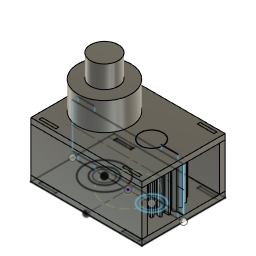
Dual Rotary Encoder Proto (Autodesk Fusion 360 design; units mm, degrees)
description: Spur Gear; Module: 0.7083333333333334; Num Teeth: 24; Pressure Angle: 20.0; Backlash: 0.00 mm
Autodesk Fusion 360 part; units mm, degrees
note: some values were not read from the file. Set by a fixed rule: which sketch regions a step uses.
sketch "BasePlate" plane through (0, 0, 0) normal (0, 0, 1) x (1, 0, 0)
  line L0 (-20, 15) -> (20, 15)
  line L1 (20, 15) -> (20, -15)
  line L2 (20, -15) -> (-20, -15)
  line L3 (-20, -15) -> (-20, 15)
  line L4 (0, 0) -> (-8.5, 0) construction
  line L5 (0, 0) -> (8.5, 0) construction
  circle A0 centre (-8.5, 0) radius 4.125
  circle A1 centre (8.5, 0) radius 4.125
  circle A2 centre (-8.5, 0) radius 7
  line L6 (-18, 14) -> (-12, 14)
  line L7 (-12, 14) -> (-12, 13)
  line L8 (-12, 13) -> (-18, 13)
  line L9 (-18, 13) -> (-18, 14)
  line L10 (18, 14) -> (12, 14)
  line L11 (12, 14) -> (12, 13)
  line L12 (12, 13) -> (18, 13)
  line L13 (18, 13) -> (18, 14)
  line L14 (18, -13) -> (12, -13)
  line L15 (12, -13) -> (12, -14)
  line L16 (12, -14) -> (18, -14)
  line L17 (18, -14) -> (18, -13)
  line L18 (-18, -13) -> (-12, -13)
  line L19 (-12, -13) -> (-12, -14)
  line L20 (-12, -14) -> (-18, -14)
  line L21 (-18, -14) -> (-18, -13)
  line L22 (-18, 13) -> (-20, 13) construction
  line L23 (-12, 14) -> (-12, 15) construction
  line L24 (12, 14) -> (12, 15) construction
  line L25 (18, 13) -> (20, 13) construction
  line L26 (-18, -13) -> (-20, -13) construction
  line L27 (-12, -14) -> (-12, -15) construction
  line L28 (12, -14) -> (12, -15) construction
  line L29 (18, -13) -> (20, -13) construction
  line L30 (0, 15) -> (0, -15)
  circle A3 centre (-8.5, 0) radius 3
  circle A4 centre (8.5, 0) radius 3
  circle A5 centre (8.5, 0) radius 4
  circle A6 centre (-8.5, 0) radius 4
  line L31 (-20, 0) -> (20, 0)
  circle A7 centre (-8.5, 0) radius 7.125
  line L32 (-17.85, 13.85) -> (-12.15, 13.85)
  line L33 (-12.15, 13.85) -> (-12.15, 13.15)
  line L34 (-12.15, 13.15) -> (-17.85, 13.15)
  line L35 (-17.85, 13.15) -> (-17.85, 13.85)
  dimension "d1" = 8.5
  dimension "d3" = 8.5
  dimension "d5" = 8.25
  dimension "d8" = 14
  dimension "d14" = 6
  dimension "d15" = 2
  dimension "d16" = 40
  dimension "d20" = 30
  dimension "d23" = 6
  dimension "d24" = 8
  dimension "d26" = 1
  dimension "d27" = 1
  dimension "d56" = 14.25
  dimension "d79" = 0.15
  constraint horizontal L0
  constraint vertical L1
  constraint horizontal L2
  constraint vertical L3
  constraint coincident L4.start L5.start
  constraint horizontal L4
  constraint coincident L4.end A0.centre
  constraint coincident L5.end A1.centre
  constraint concentric A0 A2
  constraint horizontal L6
  constraint vertical L7
  constraint horizontal L8
  constraint vertical L9
  constraint horizontal L10
  constraint vertical L11
  constraint horizontal L12
  constraint vertical L13
  constraint horizontal L14
  constraint vertical L15
  constraint horizontal L16
  constraint vertical L17
  constraint horizontal L18
  constraint vertical L19
  constraint horizontal L20
  constraint vertical L21
  constraint coincident L3 L22.end
  constraint perpendicular L3 L22
  constraint coincident L0 L23.end
  constraint perpendicular L0 L23
  constraint coincident L0 L24.end
  constraint perpendicular L0 L24
  constraint perpendicular L13 L25
  constraint coincident L3 L26.end
  constraint perpendicular L3 L26
  constraint coincident L2 L27.end
  constraint perpendicular L2 L27
  constraint coincident L2 L28.end
  constraint perpendicular L2 L28
  constraint coincident L1 L29.end
  constraint perpendicular L1 L29
  constraint coincident L0 L30.start
  constraint perpendicular L0 L30
  constraint midpoint L0 L30.start
  constraint midpoint L4.start L30
  constraint concentric A0 A3
  constraint concentric A1 A4
  constraint concentric A1 A5
  constraint concentric A0 A6
  constraint coincident L1 L25.end
  constraint equal A0 A1
  constraint equal A5 A6
  constraint equal A3 A4
  constraint equal L22 L25
  constraint equal L23 L24
  constraint equal L8 L12
  constraint midpoint L3 L31.start
  constraint midpoint L1 L31.end
  constraint midpoint L4.start L31
  constraint equal L22 L26
  constraint equal L8 L18
  constraint equal L7 L19
  constraint equal L23 L27
  constraint equal L7 L11
  constraint equal L7 L15
  constraint equal L23 L28
  constraint equal L8 L14
  constraint equal L22 L29
  constraint concentric A3 A7
  measures "d1" distance of L4.start L4.end
  measures "d3" distance of L4.start L5.end
  measures "d5" diameter of A1
  measures "d8" diameter of A2
  measures "d14" distance of L7.end L8.end
  measures "d15" distance of L8.end L22.end
  measures "d16" distance of L0.start L0.end
  measures "d20" distance of L0.start L2.end
  measures "d23" diameter of A4
  measures "d24" diameter of A5
  measures "d26" distance of L6.end L7.end
  measures "d27" distance of L6.end L23.end
  measures "d56" diameter of A7
extrude "Extrude1" add sketch "BasePlate" along normal blind 2 contours L0 L3 L30 L31 A7 | L0 L1 A1 L30 L31 | L2 L3 L30 L31 A7 | L1 L2 A1 L30 L31 | A2 L31 A7 | A2 L31 A7 | A0 A2 L31 | A0 A2 L31 makes body 1 in component "Panel Bottom"
extrude "Extrude1'" add sketch "BasePlate" along normal blind 2 separate body contours L0 L3 L30 L31 A7 | L0 L1 A1 L30 L31 | L2 L3 L30 L31 A7 | L1 L2 A1 L30 L31 makes body 2 in component "Panel Top"
move_body "Move1" bodies 2 to x (1, 0, 0) y (0, 1, 0) z (0, 0, 1) at (0, 0, 18) in component "Panel Top"
extrude "Extrude1''" add sketch "BasePlate" along normal blind 20 separate body contours A4 A5 L31 | A4 A5 L31 | A4 L31 | A4 L31 makes body 3 in component "Axle Coarse"
extrude "Extrude2" cut sketch "BasePlate" along normal blind 6 contours A4 L31 | A4 L31 bodies 3 in component "Axle Coarse"
sketch "Sketch1" plane through (0, 0, 0) normal (0, 0, 1) x (1, 0, 0) in component "Spur Gear (24 teeth)"
  circle A0 centre (0, 0) radius 7.5992
  circle A1 centre (0, 0) radius 3
extrude "Extrude1'''" add sketch "Sketch1" along normal blind 16 separate body makes body 4 in component "Spur Gear (24 teeth)"
sketch "Sketch2" plane through (0, 0, 0) normal (0, 0, 1) x (1, 0, 0) in component "Spur Gear (24 teeth)"
  spline S0 degree 5 poles (7.9616, -0.6411) (7.9652, -0.6414) (7.9722, -0.6419) (7.9828, -0.6423) (7.997, -0.6424) (8.0148, -0.6419) (8.0325, -0.6408) (8.0503, -0.6395) (8.0681, -0.6379) (8.086, -0.6363) (8.1038, -0.6345) (8.1216, -0.6326) (8.1395, -0.6304) (8.1573, -0.628) (8.1752, -0.6254) (8.193, -0.6226) (8.2109, -0.6196) (8.2287, -0.6163) (8.2466, -0.613) (8.2645, -0.6095) (8.2823, -0.6059) (8.3002, -0.6022) (8.3181, -0.5983) (8.336, -0.5942) (8.3538, -0.59) (8.3717, -0.5856) (8.3896, -0.5812) (8.4074, -0.5765) (8.4253, -0.5718) (8.4432, -0.5669) (8.461, -0.5619) (8.4789, -0.5568) (8.4968, -0.5516) (8.5146, -0.5462) (8.5325, -0.5407) (8.5503, -0.5351) (8.5681, -0.5294) (8.586, -0.5235) (8.6038, -0.5176) (8.6216, -0.5115) (8.6394, -0.5053) (8.6573, -0.499) (8.6751, -0.4926) (8.6929, -0.4861) (8.7107, -0.4795) (8.7284, -0.4728) (8.7462, -0.4659) (8.764, -0.459) (8.7817, -0.452) (8.7995, -0.4448) (8.8172, -0.4376) (8.835, -0.4302) (8.8527, -0.4228) (8.8704, -0.4152) (8.8881, -0.4076) (8.9058, -0.3998) (8.9235, -0.392) (8.9412, -0.384) (8.9588, -0.376) (8.9765, -0.3678) (8.9941, -0.3596) (9.0118, -0.3513) (9.0294, -0.3428) (9.047, -0.3343) (9.0646, -0.3257) (9.0822, -0.317) (9.0997, -0.3082) (9.1173, -0.2993) (9.1348, -0.2903) (9.1523, -0.2812) (9.1699, -0.272) (9.1839, -0.2646) (9.1944, -0.259) (9.2014, -0.2553) (9.2048, -0.2534) knots 0 0 0 0 0 0 0.01428571 0.02857143 0.04285714 0.05714286 0.07142857 0.08571429 0.1 0.11428571 0.12857143 0.14285714 0.15714286 0.17142857 0.18571429 0.2 0.21428571 0.22857143 0.24285714 0.25714286 0.27142857 0.28571429 0.3 0.31428571 0.32857143 0.34285714 0.35714286 0.37142857 0.38571429 0.4 0.41428571 0.42857143 0.44285714 0.45714286 0.47142857 0.48571429 0.5 0.51428571 0.52857143 0.54285714 0.55714286 0.57142857 0.58571429 0.6 0.61428571 0.62857143 0.64285714 0.65714286 0.67142857 0.68571429 0.7 0.71428571 0.72857143 0.74285714 0.75714286 0.77142857 0.78571429 0.8 0.81428571 0.82857143 0.84285714 0.85714286 0.87142857 0.88571429 0.9 0.91428571 0.92857143 0.94285714 0.95714286 0.97142857 0.98571429 1 1 1 1 1 1
  spline S1 degree 5 poles (7.9616, 0.6411) (7.9652, 0.6414) (7.9722, 0.6419) (7.9828, 0.6423) (7.997, 0.6424) (8.0148, 0.6419) (8.0325, 0.6408) (8.0503, 0.6395) (8.0681, 0.6379) (8.086, 0.6363) (8.1038, 0.6345) (8.1216, 0.6326) (8.1395, 0.6304) (8.1573, 0.628) (8.1752, 0.6254) (8.193, 0.6226) (8.2109, 0.6196) (8.2287, 0.6163) (8.2466, 0.613) (8.2645, 0.6095) (8.2823, 0.6059) (8.3002, 0.6022) (8.3181, 0.5983) (8.336, 0.5942) (8.3538, 0.59) (8.3717, 0.5856) (8.3896, 0.5812) (8.4074, 0.5765) (8.4253, 0.5718) (8.4432, 0.5669) (8.461, 0.5619) (8.4789, 0.5568) (8.4968, 0.5516) (8.5146, 0.5462) (8.5325, 0.5407) (8.5503, 0.5351) (8.5681, 0.5294) (8.586, 0.5235) (8.6038, 0.5176) (8.6216, 0.5115) (8.6394, 0.5053) (8.6573, 0.499) (8.6751, 0.4926) (8.6929, 0.4861) (8.7107, 0.4795) (8.7284, 0.4728) (8.7462, 0.4659) (8.764, 0.459) (8.7817, 0.452) (8.7995, 0.4448) (8.8172, 0.4376) (8.835, 0.4302) (8.8527, 0.4228) (8.8704, 0.4152) (8.8881, 0.4076) (8.9058, 0.3998) (8.9235, 0.392) (8.9412, 0.384) (8.9588, 0.376) (8.9765, 0.3678) (8.9941, 0.3596) (9.0118, 0.3513) (9.0294, 0.3428) (9.047, 0.3343) (9.0646, 0.3257) (9.0822, 0.317) (9.0997, 0.3082) (9.1173, 0.2993) (9.1348, 0.2903) (9.1523, 0.2812) (9.1699, 0.272) (9.1839, 0.2646) (9.1944, 0.259) (9.2014, 0.2553) (9.2048, 0.2534) knots 0 0 0 0 0 0 0.01428571 0.02857143 0.04285714 0.05714286 0.07142857 0.08571429 0.1 0.11428571 0.12857143 0.14285714 0.15714286 0.17142857 0.18571429 0.2 0.21428571 0.22857143 0.24285714 0.25714286 0.27142857 0.28571429 0.3 0.31428571 0.32857143 0.34285714 0.35714286 0.37142857 0.38571429 0.4 0.41428571 0.42857143 0.44285714 0.45714286 0.47142857 0.48571429 0.5 0.51428571 0.52857143 0.54285714 0.55714286 0.57142857 0.58571429 0.6 0.61428571 0.62857143 0.64285714 0.65714286 0.67142857 0.68571429 0.7 0.71428571 0.72857143 0.74285714 0.75714286 0.77142857 0.78571429 0.8 0.81428571 0.82857143 0.84285714 0.85714286 0.87142857 0.88571429 0.9 0.91428571 0.92857143 0.94285714 0.95714286 0.97142857 0.98571429 1 1 1 1 1 1
  arc A0 (9.2048, -0.2534) -> (9.2048, 0.2534) centre (0, 0) ccw
  line L0 (7.5647, -0.61) -> (7.9616, -0.6411)
  line L1 (7.5647, 0.61) -> (7.9616, 0.6411)
  line L2 (7.5647, -0.61) -> (7.5647, 0.61)
  point P0 (8.0492, -0.6395)
  point P1 (8.1374, -0.6306)
  point P2 (8.2259, -0.6168)
  point P3 (8.3147, -0.599)
  point P4 (8.4036, -0.5775)
  point P5 (8.4927, -0.5527)
  point P6 (8.5818, -0.5249)
  point P7 (8.671, -0.4941)
  point P8 (8.7602, -0.4605)
  point P9 (8.8493, -0.4242)
  point P10 (8.9384, -0.3852)
  point P11 (9.0274, -0.3438)
  point P12 (9.1162, -0.2998)
  point P13 (8.0492, 0.6395)
  point P14 (8.1374, 0.6306)
  point P15 (8.2259, 0.6168)
  point P16 (8.3147, 0.599)
  point P17 (8.4036, 0.5775)
  point P18 (8.4927, 0.5527)
  point P19 (8.5818, 0.5249)
  point P20 (8.671, 0.4941)
  point P21 (8.7602, 0.4605)
  point P22 (8.8493, 0.4242)
  point P23 (8.9384, 0.3852)
  point P24 (9.0274, 0.3438)
  point P25 (9.1162, 0.2998)
extrude "Extrude2'" add sketch "Sketch2" along normal blind 16 bodies 4 in component "Spur Gear (24 teeth)"
fillet "Fillet1" radius 0.2 2 edges at (7.5746, -0.6107, 8) (7.5746, 0.6107, 8) on bodies 4 in component "Spur Gear (24 teeth)"
pattern_circular "C-Pattern1" count 24 over 360 about axis through (0, 0, 0) along (0, 0, 1) of "Extrude2'", "Fillet1" in component "Spur Gear (24 teeth)"
sketch "Sketch3" plane through (0, 0, 0) normal (0, 0, 1) x (1, 0, 0) in component "Spur Gear (24 teeth)"
  circle A0 centre (0, 0) radius 8.5 construction
move_body "Move1'" bodies 4 to x (1, 0, 0) y (0, 1, 0) z (0, 0, 1) at (8.5, 0, 2) in component "Spur Gear (24 teeth)"
extrude "Extrude1''''" add sketch "BasePlate" along normal blind 30.5 separate body contours A3 A6 L31 | A3 A6 L31 | A3 L31 | A3 L31 makes body 5 in component "Knob Fine"
extrude "Extrude2''" cut sketch "BasePlate" along normal blind 6 contours A3 L31 | A3 L31 bodies 5 in component "Knob Fine"
extrude "Extrude1'''''" add sketch "BasePlate" along normal blind 18 separate body contours A0 A2 L31 | A0 A2 L31 makes body 6 in component "Knob Coarse"
move_body "Move1''" bodies 6 to x (1, 0, 0) y (0, 1, 0) z (0, 0, 1) at (0, 0, 2.25) in component "Knob Coarse"
sketch "Wall" plane through (0, 0, 0) normal (0, 1, 0) x (1, 0, 0)
  line L0 (20.0004, -18) -> (20.0004, -2)
  line L1 (-19.9996, -2) -> (-19.9996, -18)
  line L2 (-17.9996, 0) -> (-11.9996, 0)
  line L3 (-11.9996, 0) -> (-11.9996, -2)
  line L4 (-17.9996, -2) -> (-17.9996, 0)
  line L5 (20.0004, -2) -> (18.0004, -2)
  line L6 (18.0004, -2) -> (18.0004, 0)
  line L7 (18.0004, 0) -> (12.0004, 0)
  line L8 (12.0004, 0) -> (12.0004, -2)
  line L9 (12.0004, -2) -> (-11.9996, -2)
  line L10 (-17.9996, -2) -> (-19.9996, -2)
  line L11 (-17.9996, -18) -> (-17.9996, -20)
  line L12 (-17.9996, -20) -> (-11.9996, -20)
  line L13 (-11.9996, -20) -> (-11.9996, -18)
  line L14 (18.0004, -18) -> (18.0004, -20)
  line L15 (18.0004, -20) -> (12.0004, -20)
  line L16 (12.0004, -20) -> (12.0004, -18)
  line L17 (-17.9996, -18) -> (-19.9996, -18)
  line L18 (-11.9996, -18) -> (12.0004, -18)
  line L19 (18.0004, -18) -> (20.0004, -18)
  line L20 (-19.9996, -10) -> (20.0004, -10)
  line L21 (-19.9998, 0) -> (19.9998, 0) construction
  line L22 (0.0004, -18) -> (0, 0)
  line L23 (18.0004, -2) -> (12.0004, -2)
  line L24 (-17.9996, -2) -> (-11.9996, -2)
  line L25 (-17.9996, -18) -> (-11.9996, -18)
  line L26 (18.0004, -18) -> (12.0004, -18)
  dimension "d57" = 40
  dimension "d58" = 6
  dimension "d59" = 2
  dimension "d60" = 2
  dimension "d61" = 16
  constraint vertical L0
  constraint vertical L1
  constraint horizontal L2
  constraint vertical L3
  constraint vertical L4
  constraint perpendicular L3 L9
  constraint midpoint L1 L20.start
  constraint midpoint L0 L20.end
  constraint equal L11 L13
  constraint horizontal L18
  constraint horizontal L20
  constraint horizontal L10
  constraint horizontal L17
  constraint horizontal L12
  constraint vertical L13
  constraint vertical L16
  constraint horizontal L15
  constraint vertical L8
  constraint vertical L6
  constraint horizontal L7
  constraint horizontal L5
  constraint horizontal L19
  constraint vertical L14
  constraint equal L13 L16
  constraint equal L13 L14
  constraint equal L6 L13
  constraint equal L8 L13
  constraint equal L3 L13
  constraint equal L4 L13
  constraint equal L10 L17
  constraint equal L17 L19
  constraint equal L5 L17
  constraint equal L2 L12
  constraint equal L12 L15
  constraint equal L7 L12
  constraint midpoint L22.end L21
  constraint collinear L2 L21
  constraint midpoint L18 L22.start
  constraint coincident L22.end origin
  measures "d57" distance of L20.start L20.end
  measures "d58" distance of L11.end L12.end
  measures "d59" distance of L1.end L11.start
  measures "d60" distance of L12.end L13.end
  measures "d61" distance of L1.end L1.start
extrude "Extrude1''''''" add sketch "Wall" along normal blind 1 separate body contours L14 L15 L16 L26 | L6 L7 L8 L23 | L11 L12 L13 L25 | L2 L3 L4 L24 makes body 7 at (16.0004, 0, 1.3333) makes body 8 at (-15.9996, 0, 1.3333) makes body 9 at (14.0004, 0, 19.3333) makes body 10 at (-13.9996, 0, 18.6667) in component "Wall"
extrude "Extrude2'''" add sketch "Wall" along normal blind 2 contours L0 L18 L19 L20 L22 L26 | L0 L5 L9 L20 L22 L23 | L1 L17 L18 L20 L22 L25 | L1 L9 L10 L20 L22 L24 bodies 7 8 9 10 in component "Wall"
move_body "Move1'''" bodies 7 to x (1, 0, 0) y (0, 1, 0) z (0, 0, 1) at (0, 13, 0) in component "Wall"
mirror "Mirror1" about plane through (0, 0, 0) normal (0, 1, 0) of bodies 7 makes body 11 in component "Wall"
sketch "Sketch3 (2)" plane through (0, 0, 20.25) normal (0, 0, 1) x (-1, 0, 0)
  circle A0 centre (8.5, 0) radius 4.125
  circle A1 centre (8.5, 0) radius 7
  circle A2 centre (8.5, 0) radius 9.5
  dimension "d69" = 19
  constraint concentric A0 A2
  measures "d69" diameter of A2
extrude "Extrude2''''" add sketch "Sketch3 (2)" along normal blind 10 contours A1 | A2 bodies 6 in component "Knob Coarse"
sketch "Sketch1 (2)" plane through (0, 0, 30.5) normal (0, 0, 1) x (-1, 0, 0) in component "Knob Fine"
  circle A0 centre (8.5, 0) radius 4
  circle A1 centre (8.5, 0) radius 5
  dimension "d76" = 10
  constraint concentric A0 A1
  measures "d76" diameter of A1
extrude "Extrude3" add sketch "Sketch1 (2)" along normal blind 8 contours A0 | A1 bodies 5 in component "Knob Fine"
copy_body "CopyPasteBodies1" bodies 4 makes body 12
move_body "Move1''''" bodies 12 to x (1, 0, 0) y (0, 1, 0) z (0, 0, 1) at (-17, 0, 0)
move_body "Move2" bodies 12 to x (0.991445, 0.130526, 0) y (-0.130526, 0.991445, 0) z (0, 0, 1) at (-0.0727, 1.1095, 0)
component "Panel Bottom" placed x (1, 0, 0) y (0, 1, 0) z (0, 0, 1) at (0, 0, 0)
component "Panel Top" placed x (1, 0, 0) y (0, 1, 0) z (0, 0, 1) at (0, 0, 0)
component "Axle Coarse" placed x (1, 0, 0) y (0, 1, 0) z (0, 0, 1) at (0, 0, 0)
component "Spur Gear (24 teeth)" placed x (1, 0, 0) y (0, 1, 0) z (0, 0, 1) at (0, 0, 0)
component "Knob Fine" placed x (1, 0, 0) y (0, 1, 0) z (0, 0, 1) at (0, 0, 0)
component "Knob Coarse" placed x (1, 0, 0) y (0, 1, 0) z (0, 0, 1) at (0, 0, 0)
component "Wall" placed x (1, 0, 0) y (0, 1, 0) z (0, 0, 1) at (0, 0, 0)
equation "d1 = PointToPoint / 2"
equation "PointToPoint = 17 mm"
equation "d3 = PointToPoint / 2"
equation "LooseTol = 0.25 mm"
equation "d5 = AxleDiameter + LooseTol"
equation "AxleDiameter = 8 mm"
equation "d8 = LargeAxleDiameter"
equation "LargeAxleDiameter = 14 mm"
equation "SlotSizeX = 6 mm"
equation "SlotSizeY = 1 mm"
equation "SlotDistanceX = 2 mm"
equation "SlotDistanceY = 1 mm"
equation "d14 = SlotSizeX"
equation "d15 = SlotDistanceX"
equation "d16 = BaseWidth"
equation "BaseWidth = 40 mm"
equation "BaseDepth = 30 mm"
equation "BaseHeight = 20 mm"
equation "d20 = BaseDepth"
equation "PotShaftSize = 6 mm"
equation "d23 = PotShaftSize"
equation "d24 = AxleDiameter"
equation "d26 = SlotSizeY"
equation "d27 = SlotDistanceY"
equation "PanelThickness = 2 mm"
equation "d35 = PanelThickness"
equation "d37 = PanelThickness"
equation "d39 = BaseHeight"
equation "CutDepth = 6 mm"
equation "d42 = CutDepth"
equation "d46 = BaseHeight - PanelThickness"
equation "d47 = BaseHeight + CoarseKnobHeight + LooseTol * 2"
equation "d49 = CutDepth"
equation "d51 = BaseHeight - PanelThickness"
equation "d55 = PanelThickness + LooseTol"
equation "d56 = LargeAxleDiameter + LooseTol"
equation "d57 = BaseWidth"
equation "d58 = SlotSizeX"
equation "d59 = SlotDistanceX"
equation "d60 = PanelThickness"
equation "d61 = BaseHeight - 2 * PanelThickness"
equation "d62 = SlotSizeY"
equation "d64 = SlotSizeY + SlotDistanceY"
equation "d67 = BaseDepth / 2 - ( SlotDistanceY + SlotSizeY )"
equation "CoarseKnobDiameter = 20 mm"
equation "CoarseKnobHeight = 10 mm"
equation "FineKnobDiameter = 10 mm"
equation "FineKnobHeight = 8 mm"
equation "d74 = CoarseKnobHeight"
equation "d76 = FineKnobDiameter"
equation "d77 = FineKnobHeight"
equation "TightTol = 0.1 mm"
equation "d99 = PointToPoint / 2"
equation "d101 = PanelThickness"
equation "d102 = -PointToPoint"
